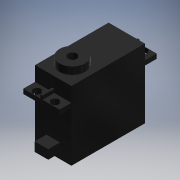
# Autodesk Inventor part: Servo
Saved by Autodesk Inventor 2017 (Build 210142000, 142)
## iProperties
Part Number: Servo
Material: Generic
Document SubType Name: Modeling
Designer: Alexander Miller
Mass: 55.2 g
Surface Area: 68.1714 cm^2
Volume: 31.271 cm^3
Density: 1.76522 g/cm^3
Appearance: Smooth - Black
s_width: 4,050 cm
s_depth: 2,000 cm
s_height: 3,800 cm
s_land: 0,650 cm
Title: Servo
Author: Alexander Miller
Autodesk Inventor part; units mm, degrees
ref_plane "YZ Plane" through (0, 0, 0) normal (1, 0, 0) x (0, 1, 0)
ref_plane "XZ Plane" through (0, 0, 0) normal (0, 1, 0) x (-1, 0, 0)
ref_plane "XY Plane" through (0, 0, 0) normal (0, 0, 1) x (1, 0, 0)
sketch "Sketch1" plane through (0, 0, 0) normal (0, 1, 0) x (-1, 0, 0)
  line L0 (-10, 20.25) -> (10, 20.25)
  line L1 (10, 20.25) -> (10, -20.25)
  line L2 (10, -20.25) -> (-10, -20.25)
  line L3 (-10, -20.25) -> (-10, 20.25)
  point P0 (0, 0)
  point P1 (0, 20.25)
  point P2 (10, 0)
  dimension "s_width" = 40.5
  dimension "s_depth" = 20
  constraints: 8 end point, 2 midpoint, 2 parallel, 1 horizontal, 1 horizontal alignment, 1 perpendicular, 1 vertical alignment
  measures "s_width" distance of L2.end L0.start
  measures "s_depth" distance of L0.start L0.end
extrude "Extrusion1" add sketch "Sketch1" along normal blind 38
sketch "Sketch2" plane through (-10, 0, 20.25) normal (0, 0, 1) x (1, 0, 0)
  line L0 (0, 38) -> (20, 38) construction
  line L1 (10, 38) -> (10, 0) construction
  line L2 (0, 27.5) -> (20, 27.5)
  line L3 (20, 27.5) -> (20, 30)
  line L4 (20, 30) -> (0, 30)
  line L5 (0, 30) -> (0, 27.5)
  dimension "d4" = 2.5
  dimension "d5" = 8
  constraints: 10 end point, 3 parallel, 1 horizontal, 1 midpoint, 1 perpendicular, 1 vertical, 1 other
  measures "d4" distance of L4.end L2.start
  measures "d5" distance between parallel lines of L4 L0
extrude "Extrusion2" add sketch "Sketch2" along normal blind 6.5 and the other way blind 47
sketch "Sketch3" plane through (-10, 30, 20.25) normal (0, 1, 0) x (1, 0, 0)
  line L0 (0, -6.5) -> (0, 0) construction
  line L1 (20, 0) -> (20, -6.5) construction
  circle A0 centre (5, -4) radius 2.25
  line L2 (0, -4) -> (20, -4) construction
  line L3 (20, -6.5) -> (0, -6.5) projected
  line L4 (0, 47) -> (0, 40.5) construction
  line L5 (0, 44.5) -> (20, 44.5) construction
  line L6 (20, 47) -> (20, 40.5) construction
  line L7 (0, 47) -> (20, 47) projected
  circle A1 centre (15, 44.5) radius 2.25
  circle A2 centre (15, -4) radius 2.25
  circle A3 centre (5, 44.5) radius 2.25
  point P0 (10, 20.25)
  dimension "d10" = 4.5
  dimension "d11" = 2.5
  dimension "d13" = 2.5
  dimension "d16" = 10
  dimension "d18" = 2.75
  constraints: 8 point on line, 4 centre point, 4 end point, 3 equal radius, 2 vertical alignment, 1 horizontal, 1 perpendicular
  measures "d10" diameter of A0
  measures "d11" distance between parallel lines of L3 L2
  measures "d13" distance between parallel lines of L5 L7
  measures "d16" distance of A2.centre A0.centre
  measures "d18" distance edge to line of A0 L0
extrude "Extrusion3" cut sketch "Sketch3" against normal up to next
sketch "Sketch4" plane through (-10, 0, 20.25) normal (0, 0, 1) x (1, 0, 0)
  line L0 (6.25, 3) -> (13.75, 3)
  line L1 (13.75, 3) -> (13.75, 8)
  line L2 (13.75, 8) -> (6.25, 8)
  line L3 (6.25, 8) -> (6.25, 3)
  line L4 (10, 0) -> (10, 27.5) construction
  line L5 (20, 27.5) -> (0, 27.5) construction
  line L6 (20, 0) -> (0, 0) construction
  point P0 (10, 8)
  dimension "d21" = 5
  dimension "d22" = 7.5
  dimension "d23" = 3
  constraints: 10 end point, 2 midpoint, 2 parallel, 1 horizontal, 1 perpendicular, 1 point on line
  measures "d21" distance of L2.end L0.start
  measures "d22" distance of L1.end L2.end
  measures "d23" distance between parallel lines of L6 L0
extrude "Extrusion4" add sketch "Sketch4" along normal up to surface (6.5 mm away)
sketch "Sketch5" plane through (-10, 38, 20.25) normal (0, 0, 1) x (1, 0, 0)
  line L0 (0, 0) -> (20, 0) construction
  line L1 (10, 0) -> (10, -8) construction
  line L2 (0, -8) -> (20, -8) construction
  line L3 (0, -8) -> (0, 0) construction
  line L4 (0, -4) -> (20, -4) construction
  line L5 (20, -8) -> (20, 0) construction
  line L6 (9.4, -8) -> (10.6, -8)
  line L7 (10.6, -8) -> (10.6, -6)
  line L8 (10.6, -6) -> (9.4, -6)
  line L9 (9.4, -6) -> (9.4, -8)
  line L10 (20, -8) -> (0, -8) projected
  point P0 (10, -38)
  dimension "d26" = 2
  dimension "d27" = 1.2
  constraints: 12 end point, 6 midpoint, 2 parallel, 1 horizontal, 1 perpendicular
  measures "d26" distance of L8.end L6.start
  measures "d27" distance of L7.end L8.end
extrude "Extrusion5" add sketch "Sketch5" against normal up to surface (53.5 mm away) from surface at 6.5
sketch "Sketch6" plane through (0, 38, 0) normal (0, 1, 0) x (1, 0, 0)
  circle A0 centre (0, -9.75) radius 7
  line L0 (0, 0) -> (0, -26.75) construction
  line L1 (-10, -26.75) -> (10, -26.75) construction
  line L2 (10, 20.25) -> (-10, 20.25) projected
  dimension "d30" = 14
  dimension "d31" = 30
  constraints: 2 end point, 1 centre point, 1 midpoint, 1 point on line
  measures "d30" diameter of A0
  measures "d31" distance from line of A0.centre L2
extrude "Extrusion6" add sketch "Sketch6" along normal blind 4
sketch "Sketch8" plane through (0, 42, 9.75) normal (0, 1, 0) x (1, 0, 0)
  circle A0 centre (0, 0) radius 2.5
  circle A1 centre (0, 0) radius 7 construction
  point P0 (0, 9.75)
  dimension "d39" = 5
  constraints: 1 centre point, 1 concentric
  measures "d39" diameter of A0
extrude "Extrusion8" cut sketch "Sketch8" against normal blind 10
equation "\"d7\" = s_land + s_width"
equation "\"s_land\" = 6.5"
body "Solid1"
